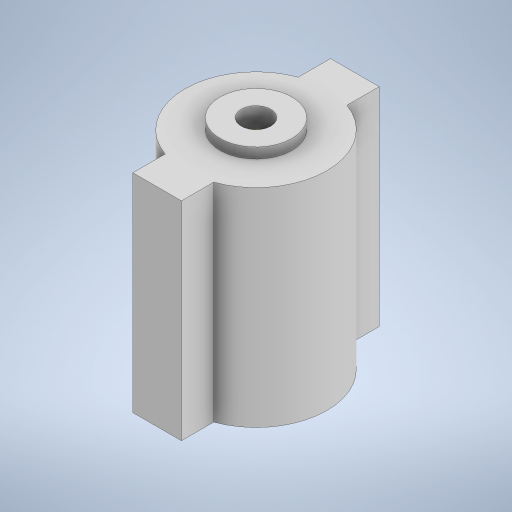
# Autodesk Inventor part: Dc Gen Outline
Saved by Autodesk Inventor 2024 (Build 280153000, 153)
## iProperties
Created: 2024-03-26
Part Number: Dc Gen Outline
Material: Generic
Document SubType Name: Modeling
Designer: albah
Density: 1 g/cm^3
Appearance: Default
Author: albah
Autodesk Inventor part; units mm, degrees
ref_plane "YZ Plane" through (0, 0, 0) normal (1, 0, 0) x (0, 1, 0)
ref_plane "XZ Plane" through (0, 0, 0) normal (0, 1, 0) x (-1, 0, 0)
ref_plane "XY Plane" through (0, 0, 0) normal (0, 0, 1) x (1, 0, 0)
sketch "Sketch1" plane through (0, 0, 0) normal (0, 1, 0) x (-1, 0, 0)
  circle A0 centre (0, 0) radius 22.6
  dimension "d0" = 45.2
  constraints: 1 centre point, 1 coincident
  measures "d0" diameter of A0
extrude "Extrusion1" add sketch "Sketch1" along normal blind 66.2
sketch "Sketch2" plane through (0, 66.2, 0) normal (0, 1, 0) x (1, 0, 0)
  circle A0 centre (0, 0) radius 11.45
  dimension "d3" = 22.9
  constraints: 1 centre point, 1 coincident
  measures "d3" diameter of A0
extrude "Extrusion2" add sketch "Sketch2" along normal blind 3.3
sketch "Sketch4" plane through (0, 0, 0) normal (0, -1, 0) x (1, 0, 0)
  circle A0 centre (0, 0) radius 12.9
  dimension "d14" = 25.8
  constraints: 1 centre point, 1 coincident
  measures "d14" diameter of A0
extrude "Extrusion3" add sketch "Sketch4" along normal blind 6.8
sketch "Sketch5" plane through (0, 69.5, 0) normal (0, 1, 0) x (1, 0, 0)
  point P0 (0, 0)
hole "Hole2" at (0, 69.5, 0) direction (0, -1, 0) diameter 9.4 depth 92.25 tip angle 118
sketch "Sketch6" plane through (0, 66.2, 0) normal (0, 1, 0) x (1, 0, 0)
  circle A0 centre (0, 0) radius 4.7 projected
  circle A1 centre (0, 0) radius 22.6 projected
  line L0 (0, 31.5) -> (7.75, 31.5)
  line L1 (0, 31.5) -> (-7.75, 31.5)
  line L2 (-7.75, 31.5) -> (-7.75, 21.2296)
  line L3 (7.75, 31.5) -> (7.75, 21.2296)
  line L4 (0, -31.5) -> (7.75, -31.5)
  line L5 (0, -31.5) -> (-7.75, -31.5)
  line L6 (-7.75, -31.5) -> (-7.75, -21.2296)
  line L7 (7.75, -31.5) -> (7.75, -21.2296)
  dimension "d25" = 7.75
  dimension "d26" = 7.75
  constraints: 16 end point, 4 point on circle, 3 perpendicular, 2 horizontal, 2 parallel, 1 point on line
  measures "d25" distance of L0.start L0.end
  measures "d26" distance of L0.start L1.end
sketch "Sketch7" plane through (0, 66.2, 0) normal (0, 1, 0) x (1, 0, 0)
  point P0 (0, 0)
extrude "Extrusion4" add sketch "Sketch6" against normal blind 66.2 contours A1 L2 L1 L0 L3 | L7 L4 L5 L6 A1
equation "\"d27\" = d1"
equation "\"d1\" = 66.2"
body "Solid1"
